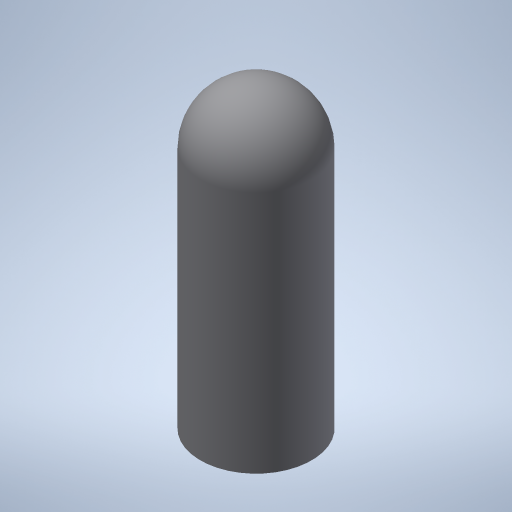
# Autodesk Inventor part: continuacion indice
Saved by Autodesk Inventor 2023 (Build 270158000, 158)
## iProperties
Created: 2022-10-21
Part Number: continuacion indice
Material: Generic
Document SubType Name: Modeling
Designer: Xiaba
Density: 1 g/cm^3
Appearance: Default
Author: Xiaba
Autodesk Inventor part; units mm, degrees
ref_plane "YZ Plane" through (0, 0, 0) normal (1, 0, 0) x (0, 1, 0)
ref_plane "XZ Plane" through (0, 0, 0) normal (0, 1, 0) x (-1, 0, 0)
ref_plane "XY Plane" through (0, 0, 0) normal (0, 0, 1) x (1, 0, 0)
sketch "Sketch1" plane through (0, 0, 0) normal (0, 1, 0) x (-1, 0, 0)
  circle A0 centre (0, 0) radius 0.875
  circle A1 centre (0, 0) radius 0.825
  dimension "d0" = 1.75
  dimension "d1" = 1.65
  constraints: 2 centre point, 2 coincident
  measures "d0" diameter of A0
  measures "d1" diameter of A1
extrude "Extrusion1" add sketch "Sketch1" along normal blind 4.7 contours A0 | A1
sketch "Sketch2" plane through (0, 0, 0) normal (1, 0, 0) x (0, 1, 0)
  circle A0 centre (1.1545, 0) radius 0.3395
  line L0 (0, 0.875) -> (4.7, 0.875) projected
  line L1 (0, -0.875) -> (4.7, -0.875) projected
  line L2 (4.7, -0.875) -> (4.7, 0.875) projected
  line L3 (4.7, 0.4277) -> (3.8411, 0.4277)
  line L4 (3.825, 0) -> (3.825, -0.875)
  arc A1 (3.825, -0.875) -> (3.825, 0.875) centre (3.825, 0) ccw
  line L5 (4.7, 0.875) -> (3.825, 0.875)
  line L6 (3.825, 0.875) -> (3.825, -0.875)
  line L7 (3.825, -0.875) -> (4.7, -0.875)
  line L8 (4.7, -0.875) -> (4.7, 0.875)
  line L9 (4.7, 0) -> (2.7552, 0)
  point P0 (0, 0)
  point P1 (4.7, 0)
  dimension "d4" = 0.679
  constraints: 14 end point, 3 perpendicular, 3 point on line, 2 centre point, 2 horizontal, 2 parallel, 2 point on circle, 1 midpoint, 1 tangent
  measures "d4" diameter of A0
revolve "Revolution1" cut sketch "Sketch2" angle 360 about axis through (0, 4.7, 0) along (0, -1, 0) contours L0 L2 L3 A1 | L3 L2 A1
shell "Shell1" thickness 0.1 removed faces 1 at (-0.3358, 0, 0.0232)
body "Solid1"
